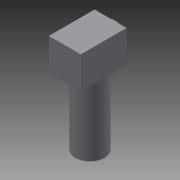
# Autodesk Inventor part: Neck_v2
Saved by Autodesk Inventor 2013 (Build 170138000, 138)
## iProperties
Created: 2012-11-28
Part Number: Neck_v2
Material: Generic
Document SubType Name: Modeling
Designer: Joe
Density: 1 g/cm^3
Author: Joe
Autodesk Inventor part; units mm, degrees
ref_plane "YZ Plane" through (0, 0, 0) normal (1, 0, 0) x (0, 1, 0)
ref_plane "XZ Plane" through (0, 0, 0) normal (0, 1, 0) x (-1, 0, 0)
ref_plane "XY Plane" through (0, 0, 0) normal (0, 0, 1) x (1, 0, 0)
sketch "Sketch1" plane through (0, 0, 0) normal (0, 1, 0) x (-1, 0, 0)
  circle A0 centre (0, 0) radius 19.25
  dimension "d0" = 38.5
  constraints: 1 centre point, 1 coincident
  measures "d0" diameter of A0
extrude "Extrusion1" add sketch "Sketch1" along normal blind 93
sketch "Sketch2" plane through (0, 93, 0) normal (0, 1, 0) x (1, 0, 0)
  circle A0 centre (0, 0) radius 19.25 projected
  line L0 (0, 0) -> (33, 0) construction
  line L1 (33, 0) -> (0, 0) construction
  line L2 (0, 0) -> (0, 21) construction
  line L3 (0, 21) -> (33, 21)
  line L4 (33, 21) -> (33, 0)
  line L5 (0, -21) -> (33, -21)
  line L6 (33, -21) -> (33, 0)
  line L7 (0, 21) -> (-33, 21)
  line L8 (-33, 21) -> (-33, 0)
  line L9 (0, -21) -> (-33, -21)
  line L10 (-33, -21) -> (-33, 0)
  dimension "d4" = 33
  dimension "d5" = 21
  constraints: 22 end point, 5 symmetric about line, 3 perpendicular, 1 collinear, 1 horizontal
  measures "d4" distance of L0.start L0.end
  measures "d5" distance of L0.start L2.end
extrude "Extrusion2" add sketch "Sketch2" along normal blind 42 contours A0 | L3 L4 L6 L5 L9 L10 L8 L7
sketch "Sketch3" plane through (33, 93, 21) normal (1, 0, 0) x (0, 0, -1)
  line L0 (0, 0) -> (42, 0) projected
  line L1 (42, 0) -> (42, 42) projected
  line L2 (0, 42) -> (42, 42) projected
  line L3 (0, 0) -> (0, 42) projected
  line L4 (0, 42) -> (42, 0) construction
  circle A0 centre (21, 21) radius 16
  point P0 (21, -93)
  dimension "d8" = 32
  constraints: 2 end point, 1 centre point, 1 midpoint
  measures "d8" diameter of A0
extrude "Extrusion3" cut sketch "Sketch3" against normal blind 6
move or copy body "Move Body2" bodies to move or copy 1 copy no rotation origin (0, 0, 0) rotation axis (1, 0, 0) rotation angle 90
move or copy body "Move Body4" bodies to move or copy 1 copy no rotation origin (0, 0, 0) rotation axis (0, 0, 1) rotation angle 90
body "Solid1"
